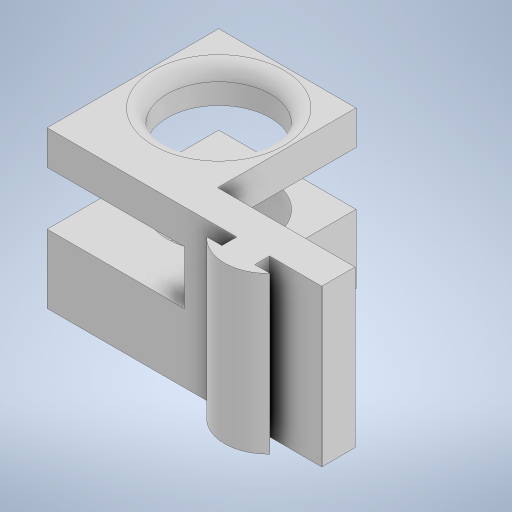
# Autodesk Inventor part: Connector MiniTec
Saved by Autodesk Inventor 2024 (Build 280153000, 153)
## iProperties
Created: 2024-01-18
Part Number: Connector MiniTec
Material: Generisch
Document SubType Name: Modeling
Designer: mariu
Density: 1 g/cm^3
Appearance: Vorgabe
Author: mariu
Autodesk Inventor part; units mm, degrees
ref_plane "YZ Plane" through (0, 0, 0) normal (1, 0, 0) x (0, 1, 0)
ref_plane "XZ Plane" through (0, 0, 0) normal (0, 1, 0) x (-1, 0, 0)
ref_plane "XY Plane" through (0, 0, 0) normal (0, 0, 1) x (1, 0, 0)
sketch "Skizze2" plane through (0, 0, 0) normal (0, 0, 1) x (1, 0, 0)
  line L0 (2.4, 0) -> (2.4, 7)
  line L1 (-2.4, 0) -> (-2.4, 7)
  line L2 (0, 0) -> (2.4, 0) construction
  line L3 (-2.4, 7) -> (2.4, 7)
  line L4 (-2.4, 0) -> (-4.6, 0)
  line L5 (2.4, 0) -> (4.6, 0)
  arc A0 (-4.6, 0) -> (4.6, 0) centre (0, 4.29) ccw
  point P0 (0, -2)
  dimension "d0" = 7
  dimension "d1" = 4.8
  dimension "d2" = 2.4
  dimension "d3" = 2.2
  dimension "d4" = 2
  constraints: 12 end point, 3 horizontal, 3 point on circle, 2 equal length, 2 vertical, 1 centre point, 1 parallel, 1 vertical alignment
  measures "d0" distance of L0.start L0.end
  measures "d1" distance between parallel lines of L1 L0
  measures "d2" distance of L2.start L0.start
  measures "d3" distance of L0.start L5.end
  measures "d4" distance of L2.start point (0, -2)
extrude "Extrusion1" add sketch "Skizze2" along normal blind 5
sketch "Skizze3" plane through (0, 0, 5) normal (0, 0, 1) x (1, 0, 0)
  line L0 (-2.4, 0) -> (-2.4, 2.2) construction
  line L1 (-2.4, 2.2) -> (-10, 2.2)
  line L2 (-2.4, 2.2) -> (10, 2.2)
  line L3 (-10, 2.2) -> (10, 2.2)
  line L4 (10, 2.2) -> (10, 7)
  line L5 (10, 7) -> (-10, 7)
  line L6 (-10, 7) -> (-10, 2.2)
  point P0 (0, 0)
  point P1 (2.4, 7)
  dimension "d7" = 2.2
  dimension "d8" = 20
  dimension "d9" = 10
  dimension "d10" = 20
  constraints: 14 end point, 3 horizontal, 2 parallel, 1 horizontal alignment, 1 perpendicular, 1 vertical alignment
  measures "d7" distance of L0.start L0.end
  measures "d8" distance of L2.end L1.end
  measures "d9" horizontal distance of point (0, 0) L2.end
  measures "d10" distance between parallel lines of L6 L4
extrude "Extrusion2" add sketch "Skizze3" against normal blind 5
sketch "Skizze5" plane through (-10, 2.2, 5) normal (-1, 0, 0) x (0, 0, 1)
  line L0 (0, 4.8) -> (-5, 4.8) projected
  line L1 (-5, 4.8) -> (0, 4.8)
  line L2 (0, 4.8) -> (0, -0.0545)
  line L3 (0, -0.0545) -> (-5, -0.0545)
  line L4 (-5, -0.0545) -> (-5, 4.8)
  point P0 (-5, -2.2)
  constraints: 8 end point, 3 perpendicular, 1 horizontal
extrude "Extrusion3" add sketch "Skizze5" along normal blind 5
sketch "Skizze6" plane through (-10, 2.1455, 0) normal (0, -1, 0) x (1, 0, 0)
  line L0 (0, 5) -> (7.6, 5) projected
  line L1 (0, 5) -> (-5, 5) projected
  line L2 (0, 5) -> (-5, 5)
  line L3 (-5, 5) -> (-5, 0)
  line L4 (-5, 0) -> (0, 0)
  line L5 (0, 0) -> (0, 5)
  point P0 (10, 0)
  constraints: 8 end point, 3 perpendicular, 1 collinear
extrude "Extrusion4" add sketch "Skizze6" against normal blind 25
sketch "Skizze12" plane through (-15, 2.2, 5) normal (-1, 0, 0) x (0, 0, 1)
  line L0 (0, -0.0545) -> (0, 24.9455) projected
  line L1 (-5, -0.0545) -> (-5, 24.9455) projected
  line L2 (0, -0.0545) -> (-5, -0.0545)
  line L3 (-5, -0.0545) -> (-5, 24.9455)
  line L4 (-5, 24.9455) -> (0, 24.9455)
  line L5 (0, 24.9455) -> (0, -0.0545)
  point P0 (-5, -2.2)
  constraints: 8 end point, 2 parallel, 1 horizontal, 1 perpendicular
extrude "Extrusion9" add sketch "Skizze12" along normal blind 15
sketch "Skizze13" plane through (0, 0, 5) normal (0, 0, 1) x (1, 0, 0)
  circle A0 centre (-20, 17.1455) radius 7.5
  line L0 (-10, 27.1455) -> (-30, 27.1455) projected
  line L1 (-30, 2.1455) -> (-30, 27.1455) projected
  point P0 (0, 0)
  point P1 (-20, 27.1455)
  dimension "d31" = 15
  dimension "d32" = 10
  dimension "d33" = 10
  constraints: 1 centre point, 1 midpoint
  measures "d31" diameter of A0
  measures "d32" distance of point (-20, 27.146) A0.centre
  measures "d33" distance from line of L1 A0.centre
extrude "Extrusion10" cut sketch "Skizze13" against normal blind 15
sketch "Skizze14" plane through (0, 0, 0) normal (0, 0, -1) x (-1, 0, 0)
  line L0 (10, 2.2) -> (10, 2.1455) projected
  line L1 (10, 2.2) -> (10, 2.1455)
  line L2 (10, 2.1455) -> (-9.9939, 2.1455)
  line L3 (-10, 2.2) -> (-2.4, 2.2) projected
  line L4 (-9.9939, 2.1455) -> (-10, 2.2)
  line L5 (-10, 2.2) -> (10, 2.2)
  point P0 (0, 0)
  constraints: 8 end point, 1 parallel, 1 perpendicular, 1 vertical
extrude "Extrusion11" add sketch "Skizze14" against normal blind 5
sketch "Skizze16" plane through (0, 0, 0) normal (0, 0, -1) x (-1, 0, 0)
  line L0 (2.4, 2.1455) -> (30, 2.1455) projected
  line L1 (30, 27.1455) -> (30, 2.1455) projected
  line L2 (10, 27.1455) -> (30, 27.1455) projected
  line L3 (10, 7) -> (10, 27.1455) projected
  line L4 (-10, 7) -> (10, 7) projected
  line L5 (-10, 7) -> (-10, 2.2) projected
  line L6 (-10, 2.2) -> (-9.9939, 2.1455) projected
  line L7 (-9.9939, 2.1455) -> (-2.4, 2.1455) projected
  line L8 (-2.4, 0) -> (-2.4, 2.1455) projected
  line L9 (-4.6, 0) -> (-2.4, 0) projected
  arc A0 (-4.6, 0) -> (4.6, 0) centre (0, 4.29) ccw projected
  line L10 (2.4, 0) -> (4.6, 0) projected
  line L11 (2.4, 2.1455) -> (2.4, 0) projected
  circle A1 centre (20, 17.1455) radius 7.5 projected
  point P0 (0, 0)
extrude "Extrusion12" add sketch "Skizze16" along normal blind 17.8
sketch "Skizze17" plane through (-10, 27.1455, 0) normal (0, 1, 0) x (1, 0, 0)
  line L0 (0, -5) -> (-20, -5) projected
  line L1 (0, -5) -> (0, 17.8) projected
  line L2 (-20, 17.8) -> (0, 17.8) projected
  line L3 (-20, -5) -> (-20, 17.8) projected
  line L4 (0, 7.8) -> (-20, 7.8)
  line L5 (-20, -5) -> (-20, 17.8) projected
  line L6 (-20, 7.8) -> (-20, 0)
  line L7 (-20, 0) -> (0, 0)
  line L8 (0, 7.8) -> (0, 0)
  point P0 (10, 0)
  dimension "d41" = 10
  dimension "d42" = 7.8
  constraints: 8 end point, 4 point on line, 2 perpendicular, 1 collinear
  measures "d41" distance between parallel lines of L2 L4
  measures "d42" distance of L4.end L6.end
extrude "Extrusion13" cut sketch "Skizze17" against normal through all contours L7 L3 L4 L1
fillet "Rundung3" radius 2 2 edges at (-27.5, 17.1455, 5) (-12.5, 17.1455, -17.8)
